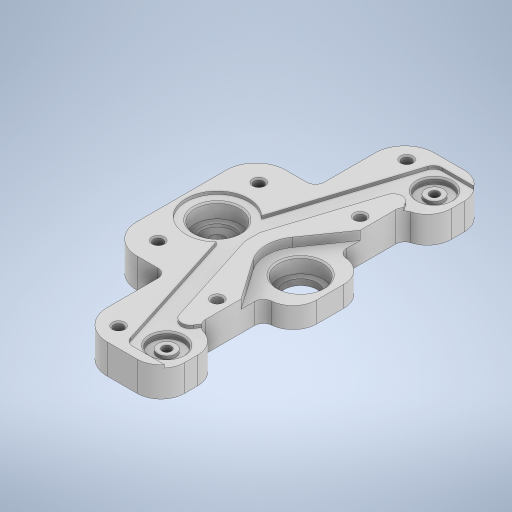
# Autodesk Inventor part: top
Saved by Autodesk Inventor 2023.1 (Build 271208000, 208)
## iProperties
Created: 2023-11-16
Part Number: top
Material: Všeobecné
Document SubType Name: Modeling
Designer: zavrel
Density: 1 g/cm^3
Appearance: Výchozí
Author: zavrel
Autodesk Inventor part; units mm, degrees
ref_plane "YZ Plane" through (0, 0, 0) normal (1, 0, 0) x (0, 1, 0)
ref_plane "XZ Plane" through (0, 0, 0) normal (0, 1, 0) x (-1, 0, 0)
ref_plane "XY Plane" through (0, 0, 0) normal (0, 0, 1) x (1, 0, 0)
sketch "Náčrt1" plane through (0, 0, 0) normal (0, 1, 0) x (-1, 0, 0)
  line L0 (-26.1298, 2.5) -> (-26.1298, 15)
  line L1 (-26.1298, 15) -> (-16.1298, 15)
  line L2 (-16.1298, 15) -> (-16.1298, 37.5)
  line L3 (-16.1298, 37.5) -> (-24.1298, 37.5)
  line L4 (-24.1298, 37.5) -> (-24.1298, 57.5)
  line L5 (-24.1298, 57.5) -> (-16.1298, 57.5)
  line L6 (-16.1298, 57.5) -> (3.8702, 57.5)
  line L7 (3.8702, 57.5) -> (3.8702, 27.5)
  line L8 (3.8702, 27.5) -> (23.8702, 27.5)
  line L9 (23.8702, 27.5) -> (23.8702, 2.5)
  line L10 (23.8702, 2.5) -> (-26.1298, 2.5) construction
  line L11 (-26.1298, 2.5) -> (-26.1298, -10)
  line L12 (-26.1298, -10) -> (-16.1298, -10)
  line L13 (-16.1298, -10) -> (-16.1298, -32.5)
  line L14 (-16.1298, -32.5) -> (-24.1298, -32.5)
  line L15 (-24.1298, -32.5) -> (-24.1298, -52.5)
  line L16 (-24.1298, -52.5) -> (-16.1298, -52.5)
  line L17 (-16.1298, -52.5) -> (3.8702, -52.5)
  line L18 (3.8702, -52.5) -> (3.8702, -22.5)
  line L19 (3.8702, -22.5) -> (23.8702, -22.5)
  line L20 (23.8702, -22.5) -> (23.8702, 2.5)
  circle A0 centre (-16.1298, 47.5) radius 5.5
  line L21 (-24.1298, 47.5) -> (17.4251, 47.5) construction
  circle A1 centre (-16.1298, -42.5) radius 5.5
  line L22 (-24.1298, -42.5) -> (17.4251, -42.5) construction
  circle A2 centre (11.8702, 2.5) radius 7.5
  circle A3 centre (-16.1298, 2.5) radius 7.5
  line L23 (-16.1298, 47.5) -> (-16.1298, -42.5) construction
  point P0 (0, 0)
  point P1 (-26.1298, 8.75)
  point P2 (-16.1298, 2.5)
  dimension "d0" = 25
  dimension "d1" = 50
  dimension "d3" = 20
  dimension "d4" = 8
  dimension "d5" = 20
  dimension "d6" = 20
  dimension "d7" = 11
  dimension "d8" = 90
  dimension "d9" = 8
  dimension "d10" = 15
  dimension "d13" = 15
  dimension "d15" = 12
  dimension "d17" = 10
  constraints: 48 end point, 12 symmetric about line, 9 perpendicular, 8 point on line, 4 centre point, 4 midpoint, 2 vertical, 1 horizontal, 1 other
  measures "d0" distance between parallel lines of L12 L1
  measures "d1" distance between parallel lines of L19 L8
  measures "d3" distance of L3.end L4.end
  measures "d4" distance between parallel lines of L13 L15
  measures "d5" distance between parallel lines of L13 L18
  measures "d6" distance between parallel lines of L18 L20
  measures "d7" diameter of A0
  measures "d8" distance of L23.end L23.start
  measures "d9" distance from line of L4 L23.start
  measures "d10" diameter of A2
  measures "d13" diameter of A3
  measures "d15" distance from line of L9 A2.centre
  measures "d17" distance of L11.end L12.end
extrude "Vysunutí1" add sketch "Náčrt1" along normal blind 10
sketch "Náčrt2" plane through (0, 0, 0) normal (0, -1, 0) x (1, 0, 0)
  line L0 (16.1298, -10) -> (16.1298, -32.5) projected
  line L1 (26.1298, -10) -> (16.1298, -10) projected
  line L2 (26.1298, 15) -> (26.1298, -10) projected
  line L3 (16.1298, 15) -> (26.1298, 15) projected
  line L4 (16.1298, 37.5) -> (16.1298, 15) projected
  line L5 (24.1298, 37.5) -> (16.1298, 37.5) projected
  line L6 (24.1298, 57.5) -> (24.1298, 37.5) projected
  line L7 (-3.8702, 57.5) -> (24.1298, 57.5) projected
  line L8 (-3.8702, 27.5) -> (-3.8702, 57.5) projected
  line L9 (-23.8702, 27.5) -> (-3.8702, 27.5) projected
  line L10 (-23.8702, -22.5) -> (-23.8702, 27.5) projected
  line L11 (-3.8702, -22.5) -> (-23.8702, -22.5) projected
  line L12 (-3.8702, -52.5) -> (-3.8702, -22.5) projected
  line L13 (24.1298, -52.5) -> (-3.8702, -52.5) projected
  line L14 (24.1298, -32.5) -> (24.1298, -52.5) projected
  line L15 (16.1298, -32.5) -> (24.1298, -32.5) projected
  circle A0 centre (16.1298, 47.5) radius 5.5 projected
  circle A1 centre (16.1298, -42.5) radius 5.5 projected
  circle A2 centre (-11.8702, 2.5) radius 7.5 projected
  circle A3 centre (16.1298, 2.5) radius 7.5 projected
  circle A4 centre (16.1298, -42.5) radius 1.5
  circle A5 centre (16.1298, 47.5) radius 5.5 projected
  circle A6 centre (16.1298, 47.5) radius 1.5
  point P0 (0, 0)
  dimension "d20" = 3
  constraints: 2 centre point, 2 coincident, 1 equal radius
  measures "d20" diameter of A6
extrude "Vysunutí2" add sketch "Náčrt2" against normal blind 8 contours A0 | A1
sketch "Náčrt3" plane through (0, 0, 0) normal (0, -1, 0) x (1, 0, 0)
  circle A0 centre (16.1298, 47.5) radius 1.5 projected
  circle A1 centre (16.1298, -42.5) radius 1.5 projected
  line L0 (16.1298, -10) -> (16.1298, -32.5) projected
  line L1 (26.1298, -10) -> (16.1298, -10) projected
  line L2 (26.1298, 15) -> (26.1298, -10) projected
  line L3 (16.1298, 15) -> (26.1298, 15) projected
  line L4 (16.1298, 37.5) -> (16.1298, 15) projected
  line L5 (24.1298, 37.5) -> (16.1298, 37.5) projected
  line L6 (24.1298, 57.5) -> (24.1298, 37.5) projected
  line L7 (-3.8702, 57.5) -> (24.1298, 57.5) projected
  line L8 (-3.8702, 27.5) -> (-3.8702, 57.5) projected
  line L9 (-23.8702, 27.5) -> (-3.8702, 27.5) projected
  line L10 (-23.8702, -22.5) -> (-23.8702, 27.5) projected
  line L11 (-3.8702, -22.5) -> (-23.8702, -22.5) projected
  line L12 (-3.8702, -52.5) -> (-3.8702, -22.5) projected
  line L13 (24.1298, -52.5) -> (-3.8702, -52.5) projected
  line L14 (24.1298, -32.5) -> (24.1298, -52.5) projected
  line L15 (16.1298, -32.5) -> (24.1298, -32.5) projected
  circle A2 centre (-11.8702, 2.5) radius 7.5 projected
  circle A3 centre (16.1298, 2.5) radius 7.5 projected
  circle A4 centre (16.1298, 2.5) radius 5.5
  point P0 (0, 0)
  dimension "d24" = 11
  constraints: 1 centre point, 1 coincident
  measures "d24" diameter of A4
extrude "Vysunutí3" add sketch "Náčrt3" against normal blind 2 contours A3
sketch "Náčrt4" plane through (0, 0, 0) normal (0, -1, 0) x (1, 0, 0)
  circle A0 centre (16.1298, 2.5) radius 5.5 projected
  circle A1 centre (16.1298, 47.5) radius 1.5 projected
  circle A2 centre (16.1298, -42.5) radius 1.5 projected
  line L0 (16.1298, -10) -> (16.1298, -32.5) projected
  line L1 (26.1298, -10) -> (16.1298, -10) projected
  line L2 (26.1298, 15) -> (26.1298, -10) projected
  line L3 (16.1298, 15) -> (26.1298, 15) projected
  line L4 (16.1298, 37.5) -> (16.1298, 15) projected
  line L5 (24.1298, 37.5) -> (16.1298, 37.5) projected
  line L6 (24.1298, 57.5) -> (24.1298, 37.5) projected
  line L7 (-3.8702, 57.5) -> (24.1298, 57.5) projected
  line L8 (-3.8702, 27.5) -> (-3.8702, 57.5) projected
  line L9 (-23.8702, 27.5) -> (-3.8702, 27.5) projected
  line L10 (-23.8702, -22.5) -> (-23.8702, 27.5) projected
  line L11 (-3.8702, -22.5) -> (-23.8702, -22.5) projected
  line L12 (-3.8702, -52.5) -> (-3.8702, -22.5) projected
  line L13 (24.1298, -52.5) -> (-3.8702, -52.5) projected
  line L14 (24.1298, -32.5) -> (24.1298, -52.5) projected
  line L15 (16.1298, -32.5) -> (24.1298, -32.5) projected
  circle A3 centre (-11.8702, 2.5) radius 7.5 projected
  circle A4 centre (-11.8702, 2.5) radius 2.5
  point P0 (0, 0)
  dimension "d27" = 5
  constraints: 1 centre point, 1 coincident
  measures "d27" diameter of A4
extrude "Vysunutí4" add sketch "Náčrt4" against normal blind 3 contours A3
sketch "Náčrt5" plane through (-11.8702, 3, 2.5) normal (0, 1, 0) x (1, 0, 0)
  circle A0 centre (0, 0) radius 7.5 projected
  circle A1 centre (0, 0) radius 2.5 projected
  circle A2 centre (0, 0) radius 2.5 projected
  circle A3 centre (0, 0) radius 5.5
  point P0 (11.8702, 2.5)
  dimension "d36" = 2
  constraints: 1 centre point, 1 coincident
  measures "d36" radial gap between concentric circles of A0 A3
extrude "Vysunutí5" add sketch "Náčrt5" along normal blind 1 contours A0
sketch "Náčrt6" plane through (16.1298, 8, -42.5) normal (0, 1, 0) x (1, 0, 0)
  circle A0 centre (0, -90) radius 5.5 projected
  circle A1 centre (0, -90) radius 1.5 projected
  circle A2 centre (0, 0) radius 5.5 projected
  circle A3 centre (0, 0) radius 1.5 projected
  circle A4 centre (0, -90) radius 1.5 projected
  circle A5 centre (0, -90) radius 3
  circle A6 centre (0, 0) radius 1.5 projected
  circle A7 centre (0, 0) radius 3
  point P0 (-16.1298, -42.5)
  dimension "d33" = 1.5
  constraints: 2 centre point, 2 coincident, 1 equal radius
  measures "d33" radial gap between concentric circles of A5 A1
extrude "Vysunutí6" cut sketch "Náčrt6" against normal blind 1 contours A0 | A2
sketch "Náčrt7" plane through (0, 10, 0) normal (0, 1, 0) x (1, 0, 0)
  line L0 (16.1298, 10) -> (16.1298, 32.5) projected
  line L1 (16.1298, 32.5) -> (24.1298, 32.5) projected
  line L2 (24.1298, 32.5) -> (24.1298, 52.5) projected
  line L3 (24.1298, 52.5) -> (-3.8702, 52.5) projected
  line L4 (-3.8702, 52.5) -> (-3.8702, 22.5) projected
  line L5 (-3.8702, 22.5) -> (-23.8702, 22.5) projected
  line L6 (-23.8702, 22.5) -> (-23.8702, -27.5) projected
  line L7 (-23.8702, -27.5) -> (-3.8702, -27.5) projected
  line L8 (-3.8702, -27.5) -> (-3.8702, -57.5) projected
  line L9 (-3.8702, -57.5) -> (24.1298, -57.5) projected
  line L10 (24.1298, -57.5) -> (24.1298, -37.5) projected
  line L11 (24.1298, -37.5) -> (16.1298, -37.5) projected
  line L12 (16.1298, -37.5) -> (16.1298, -15) projected
  line L13 (16.1298, -15) -> (26.1298, -15) projected
  line L14 (26.1298, -15) -> (26.1298, 10) projected
  line L15 (26.1298, 10) -> (16.1298, 10) projected
  circle A0 centre (16.1298, -47.5) radius 5.5 projected
  circle A1 centre (16.1298, 42.5) radius 5.5 projected
  circle A2 centre (-11.8702, -2.5) radius 7.5 projected
  circle A3 centre (16.1298, -2.5) radius 7.5 projected
  circle A4 centre (16.1298, -47.5) radius 5.5 construction
  line L16 (10.8899, -49.1715) -> (-4.7249, -0.2207) construction
  circle A5 centre (-11.8702, -2.5) radius 7.5 construction
  line L17 (-4.7249, -4.7793) -> (10.8899, 44.1715) construction
  circle A6 centre (16.1298, 42.5) radius 5.5 projected
  line L18 (12.213, -43.4476) -> (-0.0467, -5.0148)
  line L19 (16.1298, -37.5) -> (16.1298, -15) projected
  line L20 (16.1298, -37.5) -> (12.213, -43.4476)
  line L21 (24.1298, 32.5) -> (24.1298, 52.5) projected
  line L22 (24.1298, -54.5) -> (9.5373, -54.5)
  circle A7 centre (-11.8702, -2.5) radius 10.5
  line L23 (9.5373, -54.5) -> (-4.6257, -10.1005)
  line L24 (-0.0467, -2.5) -> (-0.0467, -5.0148)
  circle A8 centre (-11.8702, -2.5) radius 2.5 construction
  line L25 (-11.8702, -2.5) -> (16.1298, -2.5) construction
  line L26 (12.213, 38.4476) -> (-0.0467, 0.0148)
  line L27 (16.1298, 32.5) -> (12.213, 38.4476)
  line L28 (24.1298, 49.5) -> (9.5373, 49.5)
  line L29 (9.5373, 49.5) -> (-4.6257, 5.1005)
  line L30 (-0.0467, -2.5) -> (-0.0467, 0.0148)
  point P0 (0, 0)
  point P1 (-4.6257, 5.1005)
  dimension "d39" = 3
  dimension "d43" = 3
  dimension "d44" = 3
  constraints: 26 end point, 5 symmetric about line, 3 tangent, 2 horizontal, 2 parallel, 2 point on circle, 2 point on line, 1 vertical, 9 other
  measures "d39" distance between parallel lines of L16 L18
  measures "d43" distance between parallel lines of L9 L22
extrude "Extrusion7" cut sketch "Náčrt7" against normal blind 1 contours L27 L26 L30 L24 L18 L20 L11 L10 L22 L23 A7 L29 L28 L2 L1 | A7
sketch "Sketch8" plane through (0, 10, 0) normal (0, 1, 0) x (1, 0, 0)
  line L0 (16.1298, 32.5) -> (12.213, 38.4476) projected
  line L1 (12.213, 38.4476) -> (-0.0467, 0.0148) projected
  line L2 (-0.0467, 0.0148) -> (-0.0467, -5.0148) projected
  line L3 (-0.0467, -5.0148) -> (12.213, -43.4476) projected
  line L4 (12.213, -43.4476) -> (16.1298, -37.5) projected
  line L5 (16.1298, -37.5) -> (16.1298, -15) projected
  line L6 (16.1298, -15) -> (26.1298, -15) projected
  line L7 (26.1298, -15) -> (26.1298, 10) projected
  line L8 (26.1298, 10) -> (16.1298, 10) projected
  line L9 (16.1298, 10) -> (16.1298, 32.5) projected
  circle A0 centre (16.1298, -2.5) radius 7.5 projected
  circle A1 centre (16.1298, -2.5) radius 11.4868
  line L10 (16.1298, 10) -> (16.1298, 32.5) projected
  line L11 (16.1298, 17.5) -> (6.7265, 4.0973)
  line L12 (16.1298, -22.5) -> (6.7265, -9.0973)
  point P0 (0, 0)
  point P1 (18.102, 10)
  point P2 (18.102, -15)
  point P3 (26.1298, 3.152)
  point P4 (26.1298, -8.152)
  dimension "d49" = 20
  constraints: 4 end point, 2 point on circle, 2 point on line, 2 tangent, 1 centre point, 1 equal length
  measures "d49" distance of A0.centre L11.start
extrude "Extrusion8" cut sketch "Sketch8" against normal blind 3 contours L9 L8 L7 A1 L11 | A1 L7 | A1 L7 L6 L5 L12 | A0 picked at (25.2965, -2.5)
sketch "Sketch9" plane through (0, 10, 0) normal (0, 1, 0) x (1, 0, 0)
  line L0 (9.5373, 49.5) -> (24.1298, 49.5) projected
  line L1 (24.1298, 49.5) -> (24.1298, 52.5) projected
  line L2 (24.1298, 52.5) -> (-3.8702, 52.5) projected
  line L3 (-3.8702, 52.5) -> (-3.8702, 22.5) projected
  line L4 (-3.8702, 22.5) -> (-23.8702, 22.5) projected
  line L5 (-23.8702, 22.5) -> (-23.8702, -27.5) projected
  line L6 (-23.8702, -27.5) -> (-3.8702, -27.5) projected
  line L7 (-3.8702, -27.5) -> (-3.8702, -57.5) projected
  line L8 (-3.8702, -57.5) -> (24.1298, -57.5) projected
  line L9 (24.1298, -57.5) -> (24.1298, -54.5) projected
  line L10 (24.1298, -54.5) -> (9.5373, -54.5) projected
  line L11 (9.5373, -54.5) -> (-4.6257, -10.1005) projected
  arc A0 (-4.6257, 5.1005) -> (-4.6257, -10.1005) centre (-11.8702, -2.5) ccw projected
  line L12 (-4.6257, 5.1005) -> (9.5373, 49.5) projected
  line L13 (16.1298, -22.5) -> (6.7265, -9.0973) projected
  arc A1 (6.7265, 4.0973) -> (6.7265, -9.0973) centre (16.1298, -2.5) ccw projected
  line L14 (6.7265, 4.0973) -> (16.1298, 17.5) projected
  line L15 (16.1298, 17.5) -> (16.1298, 32.5) projected
  line L16 (16.1298, 32.5) -> (12.213, 38.4476) projected
  line L17 (12.213, 38.4476) -> (-0.0467, 0.0148) projected
  line L18 (-0.0467, 0.0148) -> (-0.0467, -5.0148) projected
  line L19 (-0.0467, -5.0148) -> (12.213, -43.4476) projected
  line L20 (12.213, -43.4476) -> (16.1298, -37.5) projected
  line L21 (16.1298, -37.5) -> (16.1298, -22.5) projected
  circle A2 centre (16.1298, -2.5) radius 7.5 projected
  line L22 (26.1298, 10) -> (26.1298, -15) projected
  line L23 (16.1298, 10) -> (26.1298, 10) projected
  line L24 (16.1298, 17.5) -> (16.1298, 10) projected
  line L25 (6.7265, 4.0973) -> (16.1298, 17.5) projected
  arc A3 (6.7265, 4.0973) -> (6.7265, -9.0973) centre (16.1298, -2.5) ccw projected
  line L26 (16.1298, -22.5) -> (6.7265, -9.0973) projected
  line L27 (16.1298, -15) -> (16.1298, -22.5) projected
  line L28 (26.1298, -15) -> (16.1298, -15) projected
  line L29 (12.213, -43.4476) -> (16.1298, -37.5) projected
  line L30 (-0.0467, -5.0148) -> (12.213, -43.4476) projected
  line L31 (-0.0467, 0.0148) -> (-0.0467, -5.0148) projected
  line L32 (12.213, 38.4476) -> (-0.0467, 0.0148) projected
  line L33 (16.1298, 32.5) -> (12.213, 38.4476) projected
  line L34 (24.1298, 32.5) -> (16.1298, 32.5) projected
  line L35 (24.1298, 49.5) -> (24.1298, 32.5) projected
  line L36 (9.5373, 49.5) -> (24.1298, 49.5) projected
  line L37 (-4.6257, 5.1005) -> (9.5373, 49.5) projected
  arc A4 (-4.6257, 5.1005) -> (-4.6257, -10.1005) centre (-11.8702, -2.5) ccw projected
  line L38 (9.5373, -54.5) -> (-4.6257, -10.1005) projected
  line L39 (24.1298, -54.5) -> (9.5373, -54.5) projected
  line L40 (24.1298, -37.5) -> (24.1298, -54.5) projected
  line L41 (16.1298, -37.5) -> (24.1298, -37.5) projected
  circle A5 centre (-11.8702, -2.5) radius 7.5 projected
  circle A6 centre (16.1298, 42.5) radius 5.5 projected
  circle A7 centre (16.1298, -47.5) radius 5.5 projected
  circle A8 centre (3.3734, -50.9251) radius 1.6
  circle A9 centre (12.1298, -26.5254) radius 1.6
  circle A10 centre (-14.8339, -19.4088) radius 1.6
  line L42 (-11.8702, -2.5) -> (16.1298, -2.5) construction
  circle A11 centre (3.3734, 45.9251) radius 1.6
  circle A12 centre (12.1298, 21.5254) radius 1.6
  circle A13 centre (-14.8339, 14.4088) radius 1.6
  point P0 (0, 0)
  dimension "d51" = 6.5749
  dimension "d52" = 7.2436
  dimension "d53" = 9.0363
  dimension "d54" = 8.0912
  dimension "d55" = 11.5254
  dimension "d56" = 4
  dimension "d57" = 3.2
  constraints: 6 centre point, 3 symmetric about line, 2 end point, 2 equal radius, 1 horizontal, 3 other
  measures "d51" distance from line of L8 A8.centre
  measures "d52" distance from line of L7 A8.centre
  measures "d53" distance from line of L5 A10.centre
  measures "d54" distance from line of L6 A10.centre
  measures "d55" distance from line of L28 A9.centre
  measures "d56" distance from line of A9.centre L21
  measures "d57" diameter of A10
extrude "Extrusion9" cut sketch "Sketch9" against normal up to surface (10 mm away) contours A8 | A9 | A10 | A11 | A12 | A13
fillet "Fillet1" radius 10 4 edges at (-23.8702, 5, 27.5) (-23.8702, 5, -22.5) (-3.8702, 5, 57.5) (-3.8702, 5, -52.5)
fillet "Fillet2" radius 3 6 edges at (16.1298, 3.5, -10) (16.1298, 4.5, -32.5) (16.1298, 3.5, 15) (16.1298, 4.5, 37.5) (-3.8702, 5, -22.5) (-3.8702, 5, 27.5)
fillet "Fillet3" radius 8 4 edges at (24.1298, 5, 57.5) (24.1298, 4.5, 37.5) (24.1298, 4.5, -32.5) (24.1298, 5, -52.5)
fillet "Fillet4" radius 8 2 edges at (26.1298, 3.5, 15) (26.1298, 3.5, -10)
fillet "Fillet5" radius 3 4 edges at (9.5373, 9.5, 54.5) (12.213, 9.5, 43.4476) (12.213, 9.5, -38.4476) (9.5373, 9.5, -49.5)
chamfer "Chamfer1" distance 0.5 angle 45 10 edges at (21.6298, 9, 47.5) (23.6298, 7, 2.5) (-4.3702, 9, 2.5) (21.6298, 9, -42.5) (1.7734, 10, 50.9251) (-16.4339, 10, 19.4088) (-16.4339, 10, -14.4088) (1.7734, 10, -45.9251) (10.5298, 10, -21.5254) (10.5298, 10, 26.5254)
sketch "Sketch10" plane through (0, 0, 0) normal (0, -1, 0) x (1, 0, 0)
  point P0 (0, 0)
